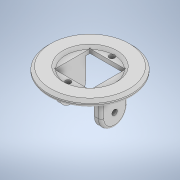
# Autodesk Inventor part: bigSpringMountB
Saved by Autodesk Inventor 2022 (Build 260153000, 153)
## iProperties
Created: 2022-03-26
Part Number: bigSpringMountB
Material: Generic
Document SubType Name: Modeling
Designer: Phabryan
Density: 1 g/cm^3
Appearance: Default
Author: Phabryan
Autodesk Inventor part; units mm, degrees
ref_plane "YZ Plane" through (0, 0, 0) normal (1, 0, 0) x (0, 1, 0)
ref_plane "XZ Plane" through (0, 0, 0) normal (0, 1, 0) x (-1, 0, 0)
ref_plane "XY Plane" through (0, 0, 0) normal (0, 0, 1) x (1, 0, 0)
sketch "Sketch1" plane through (0, 0, 0) normal (0, 1, 0) x (-1, 0, 0)
  circle A0 centre (0, 0) radius 31
  dimension "d0" = 62
  constraints: 1 centre point, 1 coincident
  measures "d0" diameter of A0
extrude "Extrusion1" add sketch "Sketch1" along normal blind 5
sketch "Sketch2" plane through (0, 5, 0) normal (0, 1, 0) x (1, 0, 0)
  circle A0 centre (0, 0) radius 20
  dimension "d3" = 40
  constraints: 1 centre point, 1 coincident
  measures "d3" diameter of A0
extrude "Extrusion2" cut sketch "Sketch2" against normal blind 2
chamfer "Chamfer1" distance 2 angle 45 1 edges at (-20, 3, 0)
sketch "Sketch3" plane through (0, 0, 0) normal (0, -1, 0) x (1, 0, 0)
  line L0 (13.2, 13.2) -> (-13.2, 13.2)
  line L1 (-13.2, 13.2) -> (-13.2, -13.2)
  line L2 (-13.2, -13.2) -> (13.2, -13.2)
  line L3 (13.2, -13.2) -> (13.2, 13.2)
  point P0 (0, 0)
  dimension "d9" = 26.4
  dimension "d10" = 26.4
  constraints: 8 end point, 2 parallel, 1 horizontal, 1 perpendicular
  measures "d9" distance of L2.end L1.end
  measures "d10" distance of L1.end L0.end
extrude "Extrusion3" cut sketch "Sketch3" against normal blind 6
sketch "Sketch4" plane through (0, 5, 0) normal (0, 1, 0) x (1, 0, 0)
  circle A0 centre (0, 16.2) radius 2
  circle A1 centre (0, -16.2) radius 2
  point P0 (0, 0)
  dimension "d13" = 4
  dimension "d14" = 4
  constraints: 2 centre point
  measures "d13" diameter of A0
  measures "d14" diameter of A1
extrude "Extrusion4" cut sketch "Sketch4" against normal blind 6
sketch "Sketch5" plane through (0, 0, 0) normal (0, -1, 0) x (1, 0, 0)
  line L0 (-13.2, -13.2) -> (-13.2, 13.2) projected
  line L1 (-13.2, 10) -> (-18.2, 10)
  line L2 (-18.2, 10) -> (-18.2, -10)
  line L3 (-18.2, -10) -> (-13.2, -10)
  line L4 (-13.2, -10) -> (-13.2, 10)
  line L5 (13.2, 13.2) -> (13.2, -13.2) projected
  line L6 (13.2, -10) -> (18.2, -10)
  line L7 (18.2, -10) -> (18.2, 10)
  line L8 (18.2, 10) -> (13.2, 10)
  line L9 (13.2, 10) -> (13.2, -10)
  point P0 (0, 0)
  dimension "d17" = 5
  dimension "d18" = 20
  dimension "d19" = 5
  dimension "d20" = 20
  constraints: 16 end point, 4 parallel, 3 point on line, 2 horizontal, 2 perpendicular
  measures "d17" distance of L3.end L2.end
  measures "d18" distance of L2.end L1.end
  measures "d19" distance of L8.end L7.end
  measures "d20" distance of L7.end L6.end
extrude "Extrusion5" add sketch "Sketch5" along normal blind 25.6
fillet "Fillet1" radius 10 4 edges at (15.7, -25.6, 10) (15.7, -25.6, -10) (-15.7, -25.6, -10) (-15.7, -25.6, 10)
fillet "Fillet2" radius 2 7 edges at (31, 0, 0) (18.2, -7.8001, 10) (18.2, -7.8001, -10) (18.2, -22.6711, 7.0711) (-18.2, -7.8001, -10) (-18.2, -7.8001, 10) (-18.2, -22.6711, -7.0711)
sketch "Sketch6" plane through (-18.2, 0, -8) normal (-1, 0, 0) x (0, 0, 1)
  circle A0 centre (8, -15.6) radius 2
  line L0 (0, 0) -> (16, 0) projected
  point P0 (8, 0)
  dimension "d25" = 4
  dimension "d31" = 15.6
  constraints: 1 centre point
  measures "d25" diameter of A0
  measures "d31" distance from line of L0 A0.centre
extrude "Extrusion6" cut sketch "Sketch6" against normal blind 50
chamfer "Chamfer2" distance 2 angle 45 1 edges at (31, 5, 0)
body "Solid1"
